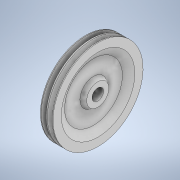
# Autodesk Inventor part: polia
Saved by Autodesk Inventor 2022.1 (Build 261234020, 234B)
## iProperties
Created: 2023-08-25
Part Number: polia
Material: Generic
Document SubType Name: Modeling
Designer: SENAI
Density: 1 g/cm^3
Appearance: Default
Author: SENAI
Autodesk Inventor part; units mm, degrees
ref_plane "YZ Plane" through (0, 0, 0) normal (1, 0, 0) x (0, 1, 0)
ref_plane "XZ Plane" through (0, 0, 0) normal (0, 1, 0) x (-1, 0, 0)
ref_plane "XY Plane" through (0, 0, 0) normal (0, 0, 1) x (1, 0, 0)
sketch "Sketch1" plane through (0, 0, 0) normal (0, 0, 1) x (1, 0, 0)
  line L0 (-0.1245, 13.5) -> (-0.1245, 23.5)
  line L1 (-0.1245, 23.5) -> (16.8755, 23.5)
  line L2 (16.8755, 23.5) -> (16.8755, 76.467)
  line L3 (16.8755, 76.467) -> (15.7439, 76.467)
  line L4 (15.7439, 76.467) -> (7.8755, 84.3355)
  line L5 (7.8755, 84.3355) -> (7.8755, 105.4051)
  line L6 (7.8755, 105.4051) -> (9.8755, 105.4051)
  line L7 (9.8755, 105.4051) -> (13.5442, 93.4051)
  line L8 (13.5442, 93.4051) -> (17.5442, 93.4051)
  line L9 (17.5442, 93.4051) -> (21.213, 105.4051)
  line L10 (21.213, 105.4051) -> (24.213, 105.4051)
  line L11 (24.213, 105.4051) -> (27.8818, 93.4051)
  line L12 (27.8818, 93.4051) -> (31.8818, 93.4051)
  line L13 (31.8818, 93.4051) -> (35.5505, 105.4051)
  line L14 (35.5505, 105.4051) -> (37.5505, 105.4051)
  line L15 (37.5505, 105.4051) -> (37.5505, 86.1513)
  line L16 (37.5505, 86.1513) -> (26.8755, 67.6615)
  line L17 (26.8755, 67.6615) -> (26.8755, 31.7281)
  line L18 (26.8755, 31.7281) -> (36.8755, 25.9546)
  line L19 (36.8755, 25.9546) -> (36.8755, 13.5)
  line L20 (36.8755, 13.5) -> (-0.1245, 13.5)
  line L21 (0, 0) -> (56.7105, 0)
  point P0 (7.8755, 94.8703)
  point P1 (16.8755, 49.9835)
  point P2 (8.3755, 23.5)
  point P3 (28.3552, 0)
  point P4 (36.8755, 19.7273)
  dimension "d0" = 27
  dimension "d1" = 17
  dimension "d3" = 8
  dimension "d4" = 2
  dimension "d5" = 107
  dimension "d6" = 107
  dimension "d7" = 3
  dimension "d8" = 12
  dimension "d9" = 107
  dimension "d10" = 2
  dimension "d11" = 4
  dimension "d12" = 4
  dimension "d13" = 10
  dimension "d14" = 45
  dimension "d15" = 30
  dimension "d16" = 47
  dimension "d17" = 60
  dimension "d18" = 155
  dimension "d19" = 10
  constraints: 44 end point, 6 point on line, 5 midpoint, 5 perpendicular, 4 parallel, 3 vertical, 1 horizontal
  measures "d0" diameter of L20 L21
  measures "d1" distance between parallel lines of L2 L0
  measures "d3" horizontal distance of L0.end point (7.875, 94.87)
  measures "d4" distance of L5.end L6.end
  measures "d5" angle of L8 L7
  measures "d6" angle of L8 L9
  measures "d7" distance of L9.end L10.end
  measures "d8" distance between parallel lines of L8 L6
  measures "d9" angle of L12 L11
  measures "d10" distance of L13.end L14.end
  measures "d11" distance of L7.end L8.end
  measures "d12" distance of L11.end L12.end
  measures "d13" distance from line of L17 point (16.875, 49.984)
  measures "d14" angle of L5 L4
  measures "d15" angle of L16 L15
  measures "d16" diameter of point (8.375, 23.5) L21
  measures "d17" angle of L19 L18
  measures "d18" diameter of L3.end point (28.355, 0)
  measures "d19" horizontal distance of L17.end point (36.875, 19.727)
revolve "Revolution1" add sketch "Sketch1" angle 360 about axis through (0, 0, 0) along (1, 0, 0)
body "Solid1"
